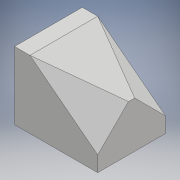
# Autodesk Inventor part: 62
Saved by Autodesk Inventor 2017 (Build 210142000, 142)
## iProperties
Part Number: 62
Material: 一般
Document SubType Name: Modeling
Designer: Brian
Density: 1 g/cm^3
Appearance: 預設
Mass: 85.1253 g
Surface Area: 114.543 cm^2
Volume: 85.1253 cm^3
Author: Brian
Autodesk Inventor part; units mm, degrees
ref_plane "YZ Plane" through (0, 0, 0) normal (1, 0, 0) x (0, 1, 0)
ref_plane "XZ Plane" through (0, 0, 0) normal (0, 1, 0) x (-1, 0, 0)
ref_plane "XY Plane" through (0, 0, 0) normal (0, 0, 1) x (1, 0, 0)
sketch "草圖1" plane through (0, 0, 0) normal (0, 1, 0) x (-1, 0, 0)
  line L0 (0, 0) -> (-54, 0)
  line L1 (-54, 0) -> (-54, -44)
  line L2 (-54, -44) -> (0, -44)
  line L3 (0, -44) -> (0, 0)
  dimension "d0" = 54
  dimension "d1" = 44
  constraints: 8 end point, 2 parallel, 1 horizontal, 1 perpendicular
  measures "d0" distance of L1.end L2.end
  measures "d1" distance of L2.end L0.start
extrude "擠出1" add sketch "草圖1" along normal mid plane 44
sketch "草圖2" plane through (0, 22, 0) normal (0, 1, 0) x (1, 0, 0)
  line L0 (0, 0) -> (54, 0) projected
  line L1 (10, 0) -> (54, 14)
  line L2 (54, 0) -> (54, 44) projected
  dimension "d4" = 10
  dimension "d5" = 30
  constraints: 2 end point, 2 point on line
  measures "d4" distance of L0.start L1.start
  measures "d5" distance of L2.end L1.end
extrude "擠出2" cut sketch "草圖2" against normal blind 60
sketch "草圖3" plane through (54, -22, -44) normal (1, 0, 0) x (0, 0, -1)
  line L0 (-30, 24) -> (-10, 44)
  line L1 (0, 44) -> (-44, 44) projected
  line L2 (-30, 44) -> (-30, 0) projected
  point P0 (-44, 22)
  point P1 (-30, 2)
  dimension "d8" = 20
  dimension "d9" = 20
  constraints: 2 end point, 2 point on line
  measures "d8" horizontal distance of L0.start L0.end
  measures "d9" horizontal distance of L0.start L0.end
ref_plane "工作平面1" through (10, 22, 0) normal (-0.4794919, -0.6205189, -0.6205189) x (0.791285, 0, -0.6114475)
sketch "草圖4" plane through (10, 22, 0) normal (-0.4794919, -0.6205189, -0.6205189) x (0.791285, 0, -0.6114475)
  line L0 (-15.1543, -12.3218) -> (93.717, -12.3218)
  line L1 (93.717, -12.3218) -> (93.717, 28.8166)
  line L2 (93.717, 28.8166) -> (-15.1543, 28.8166)
  line L3 (-15.1543, 28.8166) -> (-15.1543, -12.3218)
  point P0 (-7.9129, 13.4581)
  constraints: 8 end point, 2 parallel, 1 horizontal, 1 perpendicular
extrude "擠出3" cut sketch "草圖4" against normal blind 40
mirror "鏡射1" about plane through (0, 0, 0) normal (0, 1, 0) of "擠出3"
